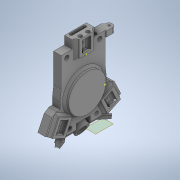
# Autodesk Inventor part: magnet holder
Saved by Autodesk Inventor 2022 (Build 260153000, 153)
## iProperties
Created: 2021-11-27
Part Number: magnet holder
Material: Polycarbonate, Clear
Document SubType Name: Modeling
Designer: alexr
Density: 1.2 g/cm^3
Appearance: Polycarbonate - Clear
Mass: 27.6489 g
Surface Area: 114.608 cm^2
Volume: 23.0407 cm^3
Author: alexr
Autodesk Inventor part; units mm, degrees
ref_plane "YZ Plane" through (0, 0, 0) normal (1, 0, 0) x (0, 1, 0)
sketch "Sketch1" plane through (0, 0, 0) normal (1, 0, 0) x (0, 1, 0)
  line L0 (-7.5, 19.95) -> (7.5, 19.95)
  line L1 (7.5, 19.95) -> (7.5, -19.95)
  line L2 (7.5, -19.95) -> (-7.5, -19.95)
  line L3 (-7.5, -19.95) -> (-7.5, 19.95)
  line L4 (-7.5, 19.95) -> (7.5, -19.95) construction
  line L5 (7.5, 19.95) -> (-7.5, -19.95) construction
  circle A0 centre (3.25, 15) radius 2
  line L6 (0, 0) -> (1.6594, 0)
  circle A1 centre (3.25, -15) radius 2
  line L7 (-7.5, 19.95) -> (-42.5, 19.95)
  line L8 (-42.5, 19.95) -> (-42.5, -19.95)
  line L9 (-42.5, -19.95) -> (-7.5, -19.95)
  line L10 (-7.5, -19.95) -> (-7.5, 19.95)
  line L11 (0, 0) -> (15, 0) construction
  line L12 (0, 0) -> (-42.5, 19.95) construction
  line L13 (0, 0) -> (-42.5, -19.95) construction
  line L14 (-42.5, 19.95) -> (-56.0784, 26.3239) construction
  line L15 (-49.0123, 11.96) -> (-58.0646, 16.2093)
  line L16 (-58.0646, 16.2093) -> (-49.5661, 34.3138)
  line L17 (-49.5661, 34.3138) -> (-40.5138, 30.0646)
  line L18 (-40.5138, 30.0646) -> (-49.0123, 11.96)
  line L19 (-49.0123, 11.96) -> (-49.5661, 34.3138) construction
  line L20 (-58.0646, 16.2093) -> (-40.5138, 30.0646) construction
  line L21 (7.5, 10) -> (15, 10)
  line L22 (15, 10) -> (15, -10)
  line L23 (15, -10) -> (7.5, -10)
  line L24 (7.5, -10) -> (7.5, 10)
  line L25 (7.5, 10) -> (15, -10) construction
  line L26 (15, 10) -> (7.5, -10) construction
  line L27 (-40.5138, 30.0646) -> (-18.9664, 19.95)
  line L28 (-42.5, -19.95) -> (-56.0784, -26.3239) construction
  line L29 (-49.0123, -11.96) -> (-58.0646, -16.2093)
  line L30 (-58.0646, -16.2093) -> (-49.5661, -34.3138)
  line L31 (-49.5661, -34.3138) -> (-40.5138, -30.0646)
  line L32 (-40.5138, -30.0646) -> (-49.0123, -11.96)
  line L33 (-49.0123, -11.96) -> (-49.5661, -34.3138) construction
  line L34 (-58.0646, -16.2093) -> (-40.5138, -30.0646) construction
  line L35 (-40.5138, -30.0646) -> (-18.9664, -19.95)
  line L36 (-58.0646, 16.2093) -> (-58.0646, -16.2093)
  line L37 (7.5, 10) -> (0, 10)
  line L38 (0, 10) -> (0, -10)
  line L39 (0, -10) -> (7.5, -10)
  line L40 (7.5, -10) -> (7.5, 10)
  point P0 (-49.2892, 23.1369)
  point P1 (11.25, 0)
  point P2 (7.5, -10)
  point P3 (7.5, 10)
  point P4 (-49.2892, -23.1369)
  dimension "d0" = 15
  dimension "d1" = 39.9
  dimension "d8" = 4
  dimension "d9" = 4.25
  dimension "d10" = 4.95
  dimension "d11" = 50
  dimension "d12" = 15
  dimension "d14" = 7.5
  dimension "d15" = 20
  dimension "d17" = 3.75
  dimension "d18" = 20
  dimension "d46" = 180
  dimension "d47" = 0
  dimension "d109" = 15
  constraints: 82 end point, 12 parallel, 9 midpoint, 8 symmetric about line, 5 horizontal, 5 perpendicular, 2 centre point, 2 point on line, 1 vertical, 1 other
  measures "d0" distance of L1.end L2.end
  measures "d1" distance of L0.end L1.end
  measures "d8" diameter of A0
  measures "d9" distance from line of L1 A0.centre
  measures "d10" distance from line of L0 A0.centre
  measures "d11" distance between parallel lines of L1 L8
  measures "d12" distance of L7.end L14.end
  measures "d14" distance from line of L11.end L1
  measures "d15" distance of L15.end L16.end
  measures "d17" distance from line of L1 point (11.25, 0)
  measures "d18" distance of L21.end L22.end
  measures "d46" angle of L12 L14
  measures "d47" distance between parallel lines of L1 L24
  measures "d109" distance between parallel lines of L22 L38
extrude "Extrusion1" add sketch "Sketch1" along normal blind 7
sketch "Sketch3" plane through (7, 0, 0) normal (1, 0, 0) x (0, 0, -1)
  line L0 (-24.7717, -37.4749) -> (-31.1455, -51.0533)
  line L1 (-31.1455, -51.0533) -> (-19.3776, -56.5774)
  line L2 (-19.3776, -56.5774) -> (-13.0037, -42.9989)
  line L3 (-13.0037, -42.9989) -> (-24.7717, -37.4749)
  line L4 (-24.7717, -37.4749) -> (-19.3776, -56.5774) construction
  line L5 (-31.1455, -51.0533) -> (-13.0037, -42.9989) construction
  line L6 (-34.3138, -49.5661) -> (-16.2093, -58.0646) projected
  line L7 (0, -10.2169) -> (0, -15.9497)
  line L8 (-6.5, 0) -> (-6.5, 15)
  line L9 (-6.5, 15) -> (6.5, 15)
  line L10 (6.5, 15) -> (6.5, 0)
  line L11 (6.5, 0) -> (-6.5, 0)
  line L12 (-6.5, 0) -> (6.5, 15) construction
  line L13 (-6.5, 15) -> (6.5, 0) construction
  line L14 (10, 7.5) -> (10, 15) projected
  line L15 (10, 15) -> (-10, 15) projected
  line L16 (-10, 15) -> (-10, 7.5) projected
  line L17 (-27.5246, -52.753) -> (-21.1508, -39.1746)
  line L18 (-21.1508, -39.1746) -> (-16.6246, -41.2992)
  line L19 (-16.6246, -41.2992) -> (-22.9985, -54.8777)
  line L20 (-22.9985, -54.8777) -> (-27.5246, -52.753)
  line L21 (-27.5246, -52.753) -> (-16.6246, -41.2992) construction
  line L22 (-21.1508, -39.1746) -> (-22.9985, -54.8777) construction
  line L23 (2.5, 0) -> (2.5, 15)
  line L24 (2.5, 15) -> (-2.5, 15)
  line L25 (-2.5, 15) -> (-2.5, 0)
  line L26 (-2.5, 0) -> (2.5, 0)
  line L27 (2.5, 0) -> (-2.5, 15) construction
  line L28 (2.5, 15) -> (-2.5, 0) construction
  line L29 (-20.3659, -52.7994) -> (-27.6077, -49.4)
  line L30 (-27.6077, -49.4) -> (-23.7834, -41.2529)
  line L31 (-23.7834, -41.2529) -> (-16.5415, -44.6523)
  line L32 (-16.5415, -44.6523) -> (-20.3659, -52.7994)
  line L33 (-20.3659, -52.7994) -> (-23.7834, -41.2529) construction
  line L34 (-27.6077, -49.4) -> (-16.5415, -44.6523) construction
  line L35 (24.7717, -37.4749) -> (31.1455, -51.0533)
  line L36 (31.1455, -51.0533) -> (19.3776, -56.5774)
  line L37 (19.3776, -56.5774) -> (13.0037, -42.9989)
  line L38 (13.0037, -42.9989) -> (24.7717, -37.4749)
  line L39 (24.7717, -37.4749) -> (19.3776, -56.5774) construction
  line L40 (31.1455, -51.0533) -> (13.0037, -42.9989) construction
  line L41 (34.3138, -49.5661) -> (16.2093, -58.0646)
  line L42 (27.5246, -52.753) -> (21.1508, -39.1746)
  line L43 (21.1508, -39.1746) -> (16.6246, -41.2992)
  line L44 (16.6246, -41.2992) -> (22.9985, -54.8777)
  line L45 (22.9985, -54.8777) -> (27.5246, -52.753)
  line L46 (27.5246, -52.753) -> (16.6246, -41.2992) construction
  line L47 (21.1508, -39.1746) -> (22.9985, -54.8777) construction
  line L48 (20.3659, -52.7994) -> (27.6077, -49.4)
  line L49 (27.6077, -49.4) -> (23.7834, -41.2529)
  line L50 (23.7834, -41.2529) -> (16.5415, -44.6523)
  line L51 (16.5415, -44.6523) -> (20.3659, -52.7994)
  line L52 (20.3659, -52.7994) -> (23.7834, -41.2529) construction
  line L53 (27.6077, -49.4) -> (16.5415, -44.6523) construction
  line L54 (4, 12) -> (-4, 12)
  line L55 (-4, 12) -> (-4, 3)
  line L56 (-4, 3) -> (4, 3)
  line L57 (4, 3) -> (4, 12)
  line L58 (4, 12) -> (-4, 3) construction
  line L59 (-4, 12) -> (4, 3) construction
  line L60 (2.5, 12) -> (4, 12)
  line L61 (4, 12) -> (4, 3)
  line L62 (4, 3) -> (2.5, 3)
  line L63 (2.5, 3) -> (2.5, 12)
  point P0 (0, 0)
  point P1 (-19.95, 7.5)
  point P2 (-22.0746, -47.0261)
  point P3 (-32.5034, -50.416)
  point P4 (-16.6131, -57.8751)
  point P5 (0, 7.5)
  point P6 (10, 20.5)
  point P7 (8, 22.5)
  point P8 (-8, 22.5)
  point P9 (22.0746, -47.0261)
  point P10 (32.5034, -50.416)
  point P11 (16.6131, -57.8751)
  point P12 (26.2499, -50.0374)
  point P13 (27.5246, -52.753)
  point P14 (21.1508, -39.1746)
  point P15 (22.4255, -41.8903)
  point P16 (17.8994, -44.0149)
  point P17 (16.6246, -41.2992)
  point P18 (22.9985, -54.8777)
  point P19 (21.7237, -52.162)
  point P20 (-22.4255, -41.8903)
  point P21 (-21.1508, -39.1746)
  point P22 (-27.5246, -52.753)
  point P23 (-26.2499, -50.0374)
  point P24 (-21.7237, -52.162)
  point P25 (-22.9985, -54.8777)
  point P26 (-16.6246, -41.2992)
  point P27 (-17.8994, -44.0149)
  point P28 (-2.5, 12)
  point P29 (-2.5, 15)
  point P30 (-2.5, 3)
  point P31 (2.5, 3)
  point P32 (2.5, 0)
  point P33 (2.5, 15)
  dimension "d48" = 15
  dimension "d49" = 13
  dimension "d50" = 0
  dimension "d51" = 0
  dimension "d52" = 15
  dimension "d53" = 13
  dimension "d54" = 0
  dimension "d55" = 20
  dimension "d56" = 3.5
  dimension "d57" = 10
  dimension "d58" = 5
  dimension "d60" = 5
  dimension "d61" = 8
  dimension "d62" = 9
  dimension "d63" = 8
  dimension "d64" = 9
  constraints: 120 end point, 18 midpoint, 17 symmetric about line, 15 parallel, 10 perpendicular, 2 point on line, 1 horizontal, 1 vertical, 1 other
  measures "d48" distance of L0.start L0.end
  measures "d49" distance of L1.end L0.end
  measures "d50" distance between parallel lines of L1 L6
  measures "d51" distance from line of point (0, 0) L7
  measures "d52" distance of L8.start L8.end
  measures "d53" distance of L8.end L9.end
  measures "d54" vertical extent of L9
  measures "d55" distance of L6.start L6.end
  measures "d56" distance from line of L6.start L0
  measures "d57" distance from line of L16 point (0, 7.5)
  measures "d58" distance of L17.end L18.end
  measures "d60" distance of L24.end L23.end
  measures "d61" distance of L29.start L29.end
  measures "d62" distance of L29.end L30.end
  measures "d63" distance of L54.start L54.end
  measures "d64" distance of L55.end L54.end
extrude "Extrusion3" add sketch "Sketch3" along normal blind 3 contours L3 L17 L31 L30 L29 L1 L0 | L3 L19 L31 L17 | L17 L29 L19 L1 | L3 L2 L1 L19 L29 L32 L31 | L8 L9 L25 L54 L55 L56 L11 | L25 L56 L23 L11 | L9 L23 L54 L25 | L23 L56 L57 L54 L9 L10 L11 | L35 L36 L42 L48 L49 L50 L38 | L42 L50 L44 L38 | L36 L44 L48 L42 | L44 L50 L51 L48 L36 L37 L38
sketch "Sketch4" plane through (7, 0, 0) normal (1, 0, 0) x (0, 0, -1)
  circle A0 centre (0, -30) radius 12.95
  line L0 (-10, 7.5) -> (-19.95, 7.5) projected
  line L1 (-16.2093, -58.0646) -> (16.2093, -58.0646) projected
  line L2 (6.5, 15) -> (-6.5, 15) projected
  point P0 (0, 0)
  dimension "d40" = 25.9
  dimension "d89" = 73.0646
  dimension "d90" = 45
  constraints: 1 centre point
  measures "d40" diameter of A0
  measures "d89" distance between parallel lines of L2 L1
  measures "d90" distance from line of A0.centre L2
extrude "Extrusion4" cut sketch "Sketch4" against normal blind 3.175
sketch "Sketch6" plane through (0, -58.0646, 16.2093) normal (0, -0.9052286, 0.4249249) x (1, 0, 0)
  circle A0 centre (7.8, 13.5) radius 1.75
  line L0 (10, 16.5) -> (10, 3.5) projected
  line L1 (7, 16.5) -> (10, 16.5) projected
  circle A1 centre (7.8, 6.5) radius 1.75
  line L2 (7, 3.5) -> (10, 3.5) projected
  line L3 (10, 16.5) -> (10, 3.5) projected
  point P0 (0, 10)
  point P1 (7, 12)
  point P2 (7, 8)
  dimension "d65" = 3.5
  dimension "d66" = 2.2
  dimension "d67" = 3
  dimension "d68" = 3.5
  dimension "d69" = 3
  dimension "d70" = 2.2
  constraints: 2 centre point, 2 other
  measures "d65" diameter of A0
  measures "d67" distance from line of L1 A0.centre
  measures "d68" diameter of A1
  measures "d69" distance from line of L2 A1.centre
extrude "Extrusion5" cut sketch "Sketch6" against normal blind 14
sketch "Sketch7" plane through (0, 15, 10) normal (0, 1, 0) x (1, 0, 0)
  circle A0 centre (7.8, 13.5) radius 1.75
  circle A1 centre (7.8, 6.5) radius 1.75
  line L0 (10, 16.5) -> (10, 3.5) projected
  line L1 (10, 16.5) -> (10, 3.5) projected
  line L2 (7, 16.5) -> (10, 16.5) projected
  line L3 (7, 3.5) -> (10, 3.5) projected
  point P0 (0, 10)
  point P1 (7, 12)
  point P2 (7, 8)
  dimension "d73" = 3.5
  dimension "d74" = 3.5
  dimension "d75" = 2.2
  dimension "d76" = 2.2
  dimension "d77" = 3
  dimension "d78" = 3
  constraints: 2 centre point, 2 other
  measures "d73" diameter of A0
  measures "d74" diameter of A1
  measures "d77" distance from line of L2 A0.centre
  measures "d78" distance from line of L3 A1.centre
extrude "Extrusion6" cut sketch "Sketch7" against normal blind 14
mirror "Mirror1" about plane through (0, 0, 0) normal (0, 0, 1) of "Extrusion5"
chamfer "Chamfer1" distance 1 angle 45 6 edges at (10, -42.9526, 20.1625) (10, -51.0997, 23.9868) (10, -51.0997, -23.9868) (10, -42.9526, -20.1625) (10, 3, 0) (10, 12, 0)
sketch "Sketch8" plane through (7, 0, 0) normal (1, 0, 0) x (0, 0, -1)
  circle A0 centre (-12.2093, -54.0646) radius 1.75
  circle A1 centre (12.2093, -54.0646) radius 1.75
  line L0 (-16.2093, -58.0646) -> (16.2093, -58.0646) projected
  point P0 (0, 0)
  dimension "d91" = 3.5
  dimension "d92" = 3.5
  dimension "d93" = 4
  dimension "d94" = 4
  dimension "d95" = 4
  dimension "d96" = 4
  constraints: 2 centre point
  measures "d91" diameter of A0
  measures "d92" diameter of A1
  measures "d93" distance from line of L0 A0.centre
  measures "d94" horizontal distance of L0.start A0.centre
  measures "d95" distance from line of L0 A1.centre
  measures "d96" horizontal distance of L0.end A1.centre
extrude "Extrusion7" cut sketch "Sketch8" against normal blind 7.75
sketch "Sketch9" plane through (7, 0, 0) normal (1, 0, 0) x (0, 0, -1)
  line L0 (-67.8204, -529.5044) -> (-67.8204, -29.5044) projected
  line L1 (-24.0204, -29.987) -> (-24.0204, -32.987) projected
  line L2 (-45.8204, -29.487) -> (-24.5204, -29.487) projected
  line L3 (-36.5634, -29.487) -> (-24.5204, -29.487) projected
  line L4 (-24.5204, -29.487) -> (-45.8204, -29.487) projected
  line L5 (-24.5204, -33.487) -> (-36.5634, -33.487) projected
  line L6 (-28.6465, -28.487) -> (-28.6465, -34.487)
  line L7 (-28.6465, -34.487) -> (-21.0204, -34.487)
  line L8 (-21.0204, -34.487) -> (-21.0204, -28.487)
  line L9 (-21.0204, -28.487) -> (-28.6465, -28.487)
  line L10 (-21.0204, -28.487) -> (-19.95, -18.9664)
  line L11 (-19.95, -18.9664) -> (-24.4191, -28.487)
  line L12 (-19.95, -18.9664) -> (-34.3138, -49.5661) projected
  point P0 (0, 0)
  point P1 (-21.0204, -31.487)
  dimension "d99" = 1
  dimension "d100" = 1
  dimension "d101" = 3
  dimension "d102" = 0
  dimension "d103" = 0
  constraints: 12 end point, 2 perpendicular, 2 point on line, 1 horizontal
  measures "d99" distance from line of L6.start L2
  measures "d100" distance from line of L5 L6.end
  measures "d101" distance from line of point (-21.02, -31.487) L1
  measures "d102" horizontal distance of L6.start L6.end
  measures "d103" distance from line of point (-21.02, -31.487) L8
extrude "Extrusion8" cut sketch "Sketch9" against normal blind 7.75
mirror "Mirror2" about plane through (0, 0, 0) normal (0, 0, 1) of "Extrusion8"
chamfer "Chamfer3" distance 3 angle 45 2 edges at (3.5, -34.487, 27.2355) (3.5, -34.487, -27.2355)
sketch "Sketch11" plane through (7, 0, 0) normal (1, 0, 0) x (0, 0, -1)
  circle A0 centre (0, -30) radius 12.95 projected
  circle A1 centre (0, -30) radius 16.95
  point P0 (0, 0)
  dimension "d110" = 4
  constraints: 1 centre point
  measures "d110" radial gap between concentric circles of A0 A1
extrude "Extrusion9" add sketch "Sketch11" along normal blind 3.175
ref_plane "Work Plane1" through (7, -30, 0) normal (1, 0, 0) x (0, 0, -1)
sketch "Sketch13" plane through (10.175, -30, 0) normal (1, 0, 0) x (0, 0, -1)
  circle A0 centre (0, 0) radius 16.95 projected
  point P0 (0, 30)
extrude "Extrusion10" add sketch "Sketch13" along normal blind 0.6
chamfer "Chamfer4" distance 2 angle 45 10 edges at (7, -30, 16.95) (7, -49.7882, 16.1906) (7, -49.7882, -16.1906) (7, -40.2369, 18.8877) (7, -44.2641, 27.9586) (7, -40.2369, -18.8877) (7, -44.2641, -27.9586) (7, 0, 0) (7, 7.5, 6.5) (7, 7.5, -6.5)
ref_plane "Work Plane2" through (3.5, 0, 0) normal (1, 0, 0) x (0, 0, -1)
sketch "Sketch15" plane through (3.5, 0, 0) normal (1, 0, 0) x (0, 0, -1)
  line L0 (-16.2093, -58.0646) -> (16.2093, -58.0646) projected
  line L1 (-7.5, 15) -> (7.5, 15)
  line L2 (7.5, 15) -> (7.5, -58.0646)
  line L3 (7.5, -58.0646) -> (-7.5, -58.0646)
  line L4 (-7.5, -58.0646) -> (-7.5, 15)
  line L5 (10, 7.5) -> (10, 15) projected
  line L6 (-10, 15) -> (-10, 7.5) projected
  line L7 (10, 15) -> (-10, 15) projected
  dimension "d124" = 15
  dimension "d125" = 20
  dimension "d126" = 2.5
  dimension "d127" = 0
  dimension "d128" = 0
  constraints: 8 end point, 2 parallel, 1 horizontal, 1 perpendicular
  measures "d124" distance of L1.start L1.end
  measures "d125" distance between parallel lines of L5 L6
  measures "d126" distance between parallel lines of L6 L4
  measures "d127" distance between parallel lines of L0 L3
  measures "d128" distance between parallel lines of L7 L1
extrude "Extrusion12" cut sketch "Sketch15" against normal blind 2.5
fillet "Fillet3" radius 1.25 4 edges at (1, -21.5323, 7.5) (1, -21.5323, -7.5) (3.5, -21.5323, -7.5) (3.5, -21.5323, 7.5)
sketch "Sketch18" plane through (0, -58.0646, -16.2093) normal (0, -1, 0) x (1, 0, 0)
  line L0 (3.5, 22.4593) -> (3.5, 9.9593) projected
  line L1 (1, 9.9593) -> (1, 22.4593) projected
  arc A0 (3.5, 22.4593) -> (1, 22.4593) centre (2.25, 22.4593) ccw projected
  line L2 (0, 32.4186) -> (0, 0) projected
  line L3 (0, 0) -> (7, 0) projected
  line L4 (7, 32.4186) -> (7, 0) projected
  line L5 (0, 32.4186) -> (7, 32.4186) projected
  arc A1 (1, 9.9593) -> (3.5, 9.9593) centre (2.25, 9.9593) ccw projected
  line L6 (0, 32.4186) -> (7, 32.4186) projected
  line L7 (2.25, 32.4186) -> (2.25, 0)
  line L8 (7, 32.4186) -> (2.25, 32.4186)
  line L9 (2.25, 32.4186) -> (2.25, 22.4186)
  line L10 (2.25, 22.4186) -> (7, 22.4186)
  line L11 (7, 22.4186) -> (7, 32.4186)
  line L12 (7, 0) -> (7, -1.3578) projected
  line L13 (7, 0) -> (2.25, 0)
  line L14 (2.25, 0) -> (2.25, 10)
  line L15 (2.25, 10) -> (7, 10)
  line L16 (7, 10) -> (7, 0)
  point P0 (0, 16.2093)
  point P1 (2.25, 23.7093)
  point P2 (2.25, 8.7093)
  point P3 (7, 10)
  point P4 (7, 22.4186)
  dimension "d142" = 10
  dimension "d143" = 10
  constraints: 18 end point, 4 parallel, 4 point on line, 3 perpendicular, 2 horizontal
  measures "d142" distance of L9.end L8.end
  measures "d143" distance of L13.end L14.end
extrude "Extrusion15" add sketch "Sketch18" along normal blind 5 contours A0 L7 L5 L4 L10 L0 | L0 L10 L7 A0 | A0 L1 A1 L7 L3 L2 L5 | L15 L4 L3 L7 A1 L0 | L0 A1 L7 L15
chamfer "Chamfer5" distance 4 distance2 5 1 edges at (7, -63.0646, 11.2093) measured on face at (6.5, -63.0646, 11.2093)
chamfer "Chamfer6" distance 4 distance2 5 1 edges at (7, -63.0646, -11.2093) measured on face at (6.5, -63.0646, -11.2093)
fillet "Fillet5" [suppressed]
sketch "Sketch20" plane through (0, -63.0646, -16.2093) normal (0, -1, 0) x (1, 0, 0)
  circle A0 centre (31, 16.2093) radius 0.2
  line L0 (1, 9.9593) -> (1, 22.4593) projected
  line L1 (31, 16.2093) -> (-3.7156, 45.0625) construction
  line L2 (7, 33.7764) -> (7, 32.4186) projected
  line L3 (7, 32.4186) -> (11.4743, 37.8019)
  line L4 (11.4743, 37.8019) -> (3.7838, 44.1938)
  line L5 (0, 32.5721) -> (0, 30.9441) projected
  line L6 (3, 32.4186) -> (0, 32.4186) projected
  line L7 (7, 32.4186) -> (0, 32.4186)
  line L8 (7, 44.7196) -> (7, 42.3584) projected
  line L9 (0, 32.4186) -> (7, 42.3584)
  point P0 (0, 16.2093)
  point P1 (6.6278, 41.83)
  dimension "d161" = 0.4
  dimension "d162" = 30
  dimension "d163" = 7
  dimension "d164" = 10
  constraints: 10 end point, 1 centre point, 1 collinear, 1 perpendicular
  measures "d161" diameter of A0
  measures "d162" distance from line of L1.start L0
  measures "d163" distance of L2.end L3.end
  measures "d164" distance of L3.end L4.end
extrude "Extrusion17" add sketch "Sketch20" against normal blind 5 contours L7 L6 L9 L4 L3
chamfer "Chamfer7" distance 3 distance2 5 1 edges at (9.2371, -63.0646, 18.901) measured on face at (8.8526, -63.0646, 19.2206)
sketch "Sketch21" plane through (0, -49.5661, 34.3138) normal (0, -0.9052286, 0.4249249) x (1, 0, 0)
  circle A0 centre (7.8, -13.5) radius 1.75 projected
  circle A1 centre (7.8, -13.5) radius 2.05
  point P0 (0, -10)
  dimension "d172" = 0.3
  constraints: 1 centre point
  measures "d172" radial gap between concentric circles of A0 A1
extrude "Extrusion18" cut sketch "Sketch21" along normal blind 21 contours A0 | A1
mirror "Mirror3" about plane through (0, 0, 0) normal (0, 0, 1) of "Extrusion17", "Extrusion18", "Chamfer7"
fillet "Fillet7" [suppressed]
fillet "Fillet8" [suppressed]
fillet "Fillet9" [suppressed]
sketch "Sketch22" plane through (0, 0, 0) normal (-1, 0, 0) x (0, 0, 1)
  line L0 (-6.25, 15) -> (-6.25, -63.0646) projected
  line L1 (6.25, -63.0646) -> (6.25, 15) projected
  line L2 (6.2093, -58.0646) -> (-6.2093, -58.0646) projected
  line L3 (6.25, 15) -> (6.25, -58.0646) projected
  line L4 (-6.2093, -58.0646) -> (6.25, -58.0646)
  line L5 (6.25, -58.0646) -> (6.25, -38.0646)
  line L6 (6.25, -38.0646) -> (-6.2093, -38.0646)
  line L7 (-6.2093, -38.0646) -> (-6.2093, -58.0646)
  line L8 (6.2093, -63.0646) -> (6.2093, -58.0646) projected
  line L9 (-6.2093, -58.0646) -> (6.2093, -58.0646)
  line L10 (6.2093, -58.0646) -> (6.2093, -63.0646)
  line L11 (6.2093, -63.0646) -> (-6.2093, -63.0646)
  line L12 (-6.2093, -63.0646) -> (-6.2093, -58.0646)
  point P0 (0, 0)
  dimension "d176" = 20
  constraints: 16 end point, 4 parallel, 2 horizontal, 2 perpendicular, 1 point on line
  measures "d176" distance of L5.end L4.end
extrude "Extrusion19" cut sketch "Sketch22" against normal blind 2
chamfer "Chamfer8" distance 1.2 angle 45 2 edges at (2.25, -60.5646, -6.2093) (2.25, -60.5646, 6.2093)
sketch "Sketch23" plane through (3.5, 0, 0) normal (-1, 0, 0) x (0, 0, 1)
  line L0 (-6.25, 15) -> (-6.25, -63.0646) projected
  line L1 (6.25, -38.0646) -> (6.25, -58.0646) projected
  line L2 (-6.25, -58.0646) -> (6.25, -58.0646)
  line L3 (6.25, -58.0646) -> (6.25, -53.0646)
  line L4 (6.25, -53.0646) -> (-6.25, -53.0646)
  line L5 (-6.25, -53.0646) -> (-6.25, -58.0646)
  line L6 (6.2093, -58.0646) -> (-6.2093, -58.0646) projected
  point P0 (0, 0)
  point P1 (-6.25, -53.0646)
  point P2 (6.25, -58.0646)
  dimension "d182" = 5
  dimension "d185" = 0
  constraints: 8 end point, 2 parallel, 2 point on line, 1 horizontal, 1 perpendicular
  measures "d182" distance of L3.end L2.end
  measures "d185" distance between parallel lines of L6 L2
extrude "Extrusion20" cut sketch "Sketch23" against normal blind 4
sketch "Sketch24" plane through (0, 0, 0) normal (0, 0, 1) x (1, 0, 0)
  line L0 (30.375, -73) -> (28.575, -73) projected
  line L1 (25.475, -73) -> (-5.7995, -54.9436)
  line L2 (0, -58.0646) -> (0, -63.0646) projected
  line L3 (3.8244, -60.5) -> (6.3244, -56.1699)
  line L4 (6.3244, -56.1699) -> (3.8244, -60.5)
  line L5 (3.8244, -60.5) -> (1.3244, -64.8301)
  line L6 (7.9894, -58.2859) -> (3.6593, -55.7859)
  line L7 (3.6593, -55.7859) -> (4.6593, -54.0538)
  line L8 (4.6593, -54.0538) -> (8.9894, -56.5538)
  line L9 (8.9894, -56.5538) -> (7.9894, -58.2859)
  line L10 (7.9894, -58.2859) -> (4.6593, -54.0538) construction
  line L11 (3.6593, -55.7859) -> (8.9894, -56.5538) construction
  point P0 (0, 0)
  point P1 (29.475, -73)
  dimension "d186" = 0
  dimension "d187" = 4
  dimension "d188" = 30
  dimension "d189" = 5
  dimension "d190" = 5
  dimension "d191" = 25
  dimension "d192" = 5
  dimension "d193" = 2
  dimension "d194" = 2.5
  dimension "d195" = 1
  constraints: 20 end point, 3 equal length, 3 perpendicular, 2 point on line, 1 midpoint
  measures "d186" distance from line of L1.start L0
  measures "d187" distance of point (29.475, -73) L1.start
  measures "d188" angle of L0 L1
  measures "d189" distance of L3.start L3.end
  measures "d190" distance of L3.start L5.end
  measures "d191" distance from line of L1.start L5
  measures "d192" distance of L6.start L6.end
  measures "d193" distance of L6.end L7.end
  measures "d194" distance from line of L9 L3.end
  measures "d195" distance from line of L3.end L8
revolve "Revolution1" add sketch "Sketch24" angle 360 about axis through (25.475, -73, 0) along (-0.8660254, 0.5, 0)
sketch "Sketch25" plane through (1.6593, -59.25, 0) normal (-0.8660254, 0.5, 0) x (0, 0, 1)
  line L0 (6.25, 17.5174) -> (6.25, 0.1969) projected
  circle A0 centre (0, 0) radius 6 projected
  line L1 (-6.2093, -4.1332) -> (-6.2093, 17.5174) projected
  line L2 (6.2093, 0.1969) -> (6.2093, -4.1332) projected
  line L3 (-10, -2) -> (10, -2)
  line L4 (10, -2) -> (10, 2)
  line L5 (10, 2) -> (-10, 2)
  line L6 (-10, 2) -> (-10, -2)
  line L7 (-10, -2) -> (10, 2) construction
  line L8 (10, -2) -> (-10, 2) construction
  line L9 (6.25, 8.0271) -> (-6.25, 8.0271) projected
  line L10 (3.8639, -5.4856) -> (7.8639, -5.4856)
  line L11 (7.8639, -5.4856) -> (7.8639, 8.0271)
  line L12 (7.8639, 8.0271) -> (3.8639, 8.0271)
  line L13 (3.8639, 8.0271) -> (3.8639, -5.4856)
  line L14 (3.8639, -5.4856) -> (7.8639, 8.0271) construction
  line L15 (7.8639, -5.4856) -> (3.8639, 8.0271) construction
  point P0 (0, 50.4824)
  point P1 (-5.6569, 2)
  point P2 (-5.6569, -2)
  point P3 (5.6569, 2)
  point P4 (5.6569, -2)
  point P5 (5.8639, 1.2707)
  point P6 (3.8639, 8.0271)
  point P7 (3.8639, 4.5902)
  point P8 (5.3552, 2.7058)
  dimension "d202" = 20
  dimension "d203" = 4
  dimension "d206" = 4
  constraints: 24 end point, 4 midpoint, 4 parallel, 2 horizontal, 2 perpendicular, 1 point on line, 2 other
  measures "d202" distance of L5.end L4.end
  measures "d203" distance of L4.end L3.end
  measures "d206" distance of L12.end L11.end
extrude "Extrusion21" [suppressed]
sketch "Sketch26" plane through (0, 0, 0) normal (-1, 0, 0) x (0, 0, 1)
  line L0 (-13.357, -93.6351) -> (11.5882, -93.6351)
  line L1 (11.5882, -93.6351) -> (11.5882, -47.8267)
  line L2 (11.5882, -47.8267) -> (-13.357, -47.8267)
  line L3 (-13.357, -47.8267) -> (-13.357, -93.6351)
  line L4 (-13.357, -93.6351) -> (11.5882, -47.8267) construction
  line L5 (11.5882, -93.6351) -> (-13.357, -47.8267) construction
  point P0 (0, 0)
  point P1 (-0.8844, -70.7309)
  constraints: 12 end point, 2 midpoint, 2 parallel, 1 horizontal, 1 perpendicular
extrude "Extrusion22" cut sketch "Sketch26" along normal blind 4
chamfer "Chamfer9" [suppressed]
sketch "Sketch27" plane through (0, 7.5, -10) normal (0, 1, 0) x (1, 0, 0)
  line L0 (8, 16) -> (8, 13.3) projected
  arc A0 (8, 16) -> (5.5, 18.5) centre (5.5, 16) ccw projected
  line L1 (4.5, 18.5) -> (5.5, 18.5) projected
  arc A1 (4.5, 18.5) -> (2, 16) centre (4.5, 16) ccw projected
  line L2 (2, 13.3) -> (2, 16) projected
  line L3 (-4, 13.3) -> (2, 13.3) projected
  line L4 (-4, 0) -> (-4, 13.3) projected
  line L5 (8, 0) -> (-4, 0) projected
  line L6 (8, 10.95) -> (8, 0) projected
  line L7 (7.7, 10.95) -> (8, 10.95) projected
  arc A2 (6.5, 12.15) -> (7.7, 10.95) centre (7.7, 12.15) ccw projected
  line L8 (6.5, 12.6) -> (6.5, 12.15) projected
  line L9 (5, 12.6) -> (6.5, 12.6) projected
  line L10 (5, 12.6) -> (5, 13.3) projected
  line L11 (8, 13.3) -> (5, 13.3) projected
  line L12 (3.45, 15.0843) -> (3.45, 16.2157) projected
  arc A3 (6.55, 16.2157) -> (3.45, 16.2157) centre (5, 15.65) ccw projected
  line L13 (6.55, 16.2157) -> (6.55, 15.0843) projected
  arc A4 (3.45, 15.0843) -> (6.55, 15.0843) centre (5, 15.65) ccw projected
  circle A5 centre (5, 2.55) radius 1.5 projected
  line L14 (0, 9.95) -> (7, 9.95) projected
  circle A6 centre (5, 15.65) radius 1
  circle A7 centre (5, 2.55) radius 1.5
  circle A8 centre (5, 2.55) radius 1.7
  line L15 (0, 9.95) -> (-0.2137, 9.95)
  line L16 (-0.2137, 9.95) -> (-0.2137, 13.3)
  line L17 (7, 9.95) -> (8, 9.95)
  line L18 (8, 9.95) -> (8, 13.3)
  point P0 (0, -10)
  dimension "d210" = 2
  dimension "d211" = 0.2
  constraints: 8 end point, 3 centre point, 3 point on line, 2 coincident, 2 perpendicular, 1 concentric, 1 horizontal
  measures "d210" diameter of A6
  measures "d211" radial gap between concentric circles of A5 A8
extrude "Extrusion23" add sketch "Sketch27" against normal blind 5 contours L0 L11 L10 L9 L8 A2 L7 L6 L17 L14 L15 L16 L3 L2 A1 L1 A0 | L18 L7 A2 L8 L9 L10 L11 | L12 A3 L13 A4
sketch "Sketch28" plane through (0, 7.5, -10) normal (0, 1, 0) x (1, 0, 0)
  line L0 (8, 16) -> (8, 13.3) projected
  arc A0 (8, 16) -> (5.5, 18.5) centre (5.5, 16) ccw projected
  line L1 (4.5, 18.5) -> (5.5, 18.5) projected
  arc A1 (4.5, 18.5) -> (2, 16) centre (4.5, 16) ccw projected
  line L2 (2, 13.3) -> (2, 16) projected
  line L3 (-4, 13.3) -> (2, 13.3) projected
  line L4 (-4, 0) -> (-4, 13.3) projected
  line L5 (8, 0) -> (-4, 0) projected
  line L6 (8, 10.95) -> (8, 0) projected
  line L7 (7.7, 10.95) -> (8, 10.95) projected
  arc A2 (6.5, 12.15) -> (7.7, 10.95) centre (7.7, 12.15) ccw projected
  line L8 (6.5, 12.6) -> (6.5, 12.15) projected
  line L9 (5, 12.6) -> (6.5, 12.6) projected
  line L10 (5, 12.6) -> (5, 13.3) projected
  line L11 (8, 13.3) -> (5, 13.3) projected
  line L12 (3.45, 15.0843) -> (3.45, 16.2157) projected
  arc A3 (6.55, 16.2157) -> (3.45, 16.2157) centre (5, 15.65) ccw projected
  line L13 (6.55, 16.2157) -> (6.55, 15.0843) projected
  arc A4 (3.45, 15.0843) -> (6.55, 15.0843) centre (5, 15.65) ccw projected
  circle A5 centre (5, 2.55) radius 1.5 projected
  circle A6 centre (5, 2.55) radius 1.7
  line L14 (0, 9.95) -> (0, 0) projected
  line L15 (-0.2137, 9.95) -> (0, 9.95) projected
  line L16 (0, 9.95) -> (0, 13.3)
  line L17 (-0.2187, 9.95) -> (-4, 9.95)
  point P0 (0, -10)
  dimension "d214" = 0.2
  constraints: 4 end point, 2 perpendicular, 2 point on line, 1 centre point
  measures "d214" radial gap between concentric circles of A5 A6
extrude "Extrusion24" cut sketch "Sketch28" against normal blind 5 contours L16 L14 L5 L4 L3 | A5 | A6
chamfer "Chamfer10" distance 2 angle 45 1 edges at (2, 5, -23.3)
sketch "Sketch29" plane through (5.9894, -61.75, 0) normal (0.8660254, -0.5, 0) x (0, 0, -1)
  circle A0 centre (0, 0) radius 6 projected
  circle A1 centre (0, 0) radius 4 projected
  point P0 (0, 50.4824)
extrude "Extrusion25" [suppressed]
ref_plane "Work Plane3" through (0, -68.0646, -16.2093) normal (0, -1, 0) x (1, 0, 0)
sketch "Sketch30" plane through (0, -68.0646, -16.2093) normal (0, -1, 0) x (1, 0, 0)
  line L0 (12.2672, 2.5378) -> (-11.7715, 2.5378)
  line L1 (-11.7715, 2.5378) -> (-11.7715, 28.4765)
  line L2 (-11.7715, 28.4765) -> (12.2672, 28.4765)
  line L3 (12.2672, 28.4765) -> (12.2672, 2.5378)
  point P0 (0, 16.2093)
  constraints: 8 end point, 2 parallel, 1 horizontal, 1 perpendicular
extrude "Extrusion26" cut sketch "Sketch30" along normal blind 6.5
sketch "Sketch31" plane through (1.6593, -59.25, 0) normal (-0.8660254, 0.5, 0) x (0, 0, 1)
  point P0 (0, 50.4824)
sketch "Sketch32" plane through (10, 0, 0) normal (1, 0, 0) x (0, 0, -1)
  point P0 (0, 0)
sketch "Sketch33" plane through (10, 0, 0) normal (1, 0, 0) x (0, 0, -1)
  circle A0 centre (0, 8) radius 0.5
  line L0 (4, 13) -> (-4, 13) projected
  line L1 (-4, 2) -> (4, 2) projected
  line L2 (4, 2) -> (4, 13) projected
  line L3 (-4, 13) -> (-4, 2) projected
  line L4 (-20.7908, -53.7046) -> (-16.1166, -43.7471) projected
  line L5 (-23.3585, -40.3477) -> (-28.0326, -50.3052) projected
  line L6 (-16.1166, -43.7471) -> (-23.3585, -40.3477) projected
  line L7 (-28.0326, -50.3052) -> (-20.7908, -53.7046) projected
  circle A1 centre (-22.0746, -47.0261) radius 0.5
  line L8 (0, -52.0049) -> (0, -49.1568)
  circle A2 centre (22.0746, -47.0261) radius 0.5
  point P0 (0, 0)
  dimension "d225" = 1
  dimension "d226" = 11
  dimension "d227" = 8
  dimension "d228" = 5.5
  dimension "d229" = 8
  dimension "d230" = 11
  dimension "d231" = 1
  dimension "d232" = 5.5
  dimension "d233" = 4
  constraints: 3 centre point, 2 end point, 1 symmetric about line, 1 vertical, 1 other
  measures "d225" diameter of A0
  measures "d226" distance between parallel lines of L0 L1
  measures "d227" distance between parallel lines of L2 L3
  measures "d228" distance edge to line of A0 L1
  measures "d229" distance between parallel lines of L4 L5
  measures "d230" distance between parallel lines of L6 L7
  measures "d231" diameter of A1
  measures "d232" distance from line of A1.centre L7
  measures "d233" distance from line of A1.centre L4
extrude "Extrusion27" cut sketch "Sketch33" against normal blind 6.5 contours A0 | A1 | A2
sketch "Sketch34" plane through (0, 0, 0) normal (-1, 0, 0) x (0, 0, 1)
  circle A0 centre (0, -30) radius 16.95 projected
  circle A1 centre (0, -30) radius 12.95
  point P0 (0, 0)
  dimension "d236" = 25.9
  constraints: 1 centre point, 1 coincident
  measures "d236" diameter of A1
extrude "Extrusion28" cut sketch "Sketch34" against normal blind 6.5 contours A1
equation "\"d17\" = 0.5 * d14"
equation "\"d53\" = d49"
equation "\"d56\" = -0.5 * d49 + 0.5 * d55"
equation "\"d69\" = d67"
equation "\"d70\" = d66"
equation "\"d76\" = d75"
equation "\"d78\" = d77"
equation "\"d94\" = d93"
equation "\"d95\" = d93"
equation "\"d96\" = d95"
equation "\"d100\" = d99"
body "Solid1"
